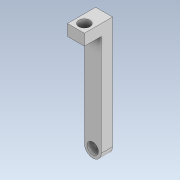
# Autodesk Inventor part: 零件2
Saved by Autodesk Inventor 2022 (Build 260153000, 153)
## iProperties
Created: 2023-04-20
Part Number: 零件2
Material: 一般
Document SubType Name: Modeling
Designer: Johnny Jou
Density: 1 g/cm^3
Appearance: 預設
Author: Johnny Jou
Autodesk Inventor part; units mm, degrees
ref_plane "YZ Plane" through (0, 0, 0) normal (1, 0, 0) x (0, 1, 0)
ref_plane "XZ Plane" through (0, 0, 0) normal (0, 1, 0) x (-1, 0, 0)
ref_plane "XY Plane" through (0, 0, 0) normal (0, 0, 1) x (1, 0, 0)
sketch "草圖1" plane through (0, 0, 0) normal (0, 0, 1) x (1, 0, 0)
  circle A0 centre (0, 0) radius 5
  line L0 (0, 0) -> (0, 100) construction
  line L1 (-7.5, 0) -> (-7.5, 100)
  line L2 (7.5, 100) -> (7.5, 0)
  arc A1 (-7.5, 0) -> (7.5, 0) centre (0, 0) ccw
  arc A2 (7.5, 100) -> (-7.5, 100) centre (0, 100) ccw
  line L3 (-7.5, 100) -> (7.5, 100)
  point P0 (0, 50)
  dimension "d0" = 10
  dimension "d1" = 15
  dimension "d2" = 100
  constraints: 10 end point, 4 point on circle, 4 tangent, 3 centre point, 1 coincident, 1 horizontal, 1 midpoint, 1 parallel, 1 vertical
  measures "d0" diameter of A0
  measures "d1" distance between parallel lines of L2 L1
  measures "d2" distance of L0.start L0.end
extrude "擠出1" add sketch "草圖1" along normal blind 10 contours L1 L3 L2 A1
sketch "草圖2" plane through (-7.5, 100, 0) normal (0, 1, 0) x (1, 0, 0)
  line L0 (15, -10) -> (0, -10) projected
  line L1 (15, -25) -> (0, -25)
  line L2 (0, -25) -> (0, -10)
  line L3 (0, -10) -> (15, -10)
  line L4 (15, -10) -> (15, -25)
  line L5 (15, -25) -> (0, -10) construction
  line L6 (0, -25) -> (15, -10) construction
  line L7 (15, 0) -> (15, -10) projected
  circle A0 centre (7.5, -17.5) radius 5
  point P0 (7.5, 0)
  point P1 (15, -10)
  dimension "d13" = 0
  dimension "d14" = 15
  dimension "d15" = 10
  constraints: 12 end point, 2 midpoint, 2 parallel, 1 centre point, 1 coincident, 1 horizontal, 1 perpendicular
  measures "d13" distance between parallel lines of L7 L4
  measures "d14" distance between parallel lines of L0 L1
  measures "d15" diameter of A0
extrude "擠出2" add sketch "草圖2" against normal blind 10
